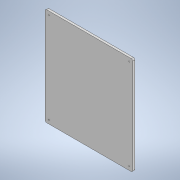
# Autodesk Inventor part: Etage 1_CPY
Saved by Autodesk Inventor 2020.1 (Build 241239000, 239)
## iProperties
Created: 2019-11-15
Part Number: Etage 1_CPY
Material: Generic
Document SubType Name: Modeling
Designer: Admin
Density: 1 g/cm^3
Appearance: Default
Author: Admin
Autodesk Inventor part; units mm, degrees
ref_plane "YZ Plane" through (0, 0, 0) normal (1, 0, 0) x (0, 1, 0)
ref_plane "XZ Plane" through (0, 0, 0) normal (0, 1, 0) x (-1, 0, 0)
ref_plane "XY Plane" through (0, 0, 0) normal (0, 0, 1) x (1, 0, 0)
sketch "Sketch1" plane through (0, 0, 0) normal (0, 0, 1) x (1, 0, 0)
  line L0 (-118.6456, 73.2494) -> (122.9544, 73.2494)
  line L1 (122.9544, 73.2494) -> (122.9544, -196.7506)
  line L2 (122.9544, -196.7506) -> (-118.6456, -196.7506)
  line L3 (-118.6456, -196.7506) -> (-118.6456, 73.2494)
  circle A0 centre (-108.6456, 63.2494) radius 1.5
  circle A1 centre (112.9544, 63.2494) radius 1.5
  circle A2 centre (-108.6456, -186.7506) radius 1.5
  circle A3 centre (112.9544, -186.7506) radius 1.5
  point P0 (0, 0)
  dimension "d0" = 241.6
  dimension "d1" = 270
  dimension "d2" = 10
  dimension "d3" = 10
  dimension "d4" = 3
  dimension "d5" = 10
  dimension "d6" = 10
  dimension "d7" = 3
  dimension "d8" = 10
  dimension "d9" = 10
  dimension "d10" = 3
  dimension "d11" = 10
  dimension "d12" = 10
  dimension "d13" = 3
  constraints: 8 end point, 4 centre point, 2 parallel, 1 horizontal, 1 perpendicular
  measures "d0" distance of L0.start L0.end
  measures "d1" distance of L0.end L1.end
  measures "d2" distance from line of L0 A0.centre
  measures "d3" distance from line of L3 A0.centre
  measures "d4" diameter of A0
  measures "d5" distance from line of L0 A1.centre
  measures "d6" distance from line of L1 A1.centre
  measures "d7" diameter of A1
  measures "d8" distance from line of L1 A3.centre
  measures "d9" distance from line of L2 A3.centre
  measures "d10" diameter of A3
  measures "d11" distance from line of L3 A2.centre
  measures "d12" distance from line of L2 A2.centre
  measures "d13" diameter of A2
extrude "Extrusion1" add sketch "Sketch1" along normal blind 6
fillet "Fillet1" radius 4 4 edges at (-118.6456, 73.2494, 3) (122.9544, 73.2494, 3) (122.9544, -196.7506, 3) (-118.6456, -196.7506, 3)
body "Solid1"
